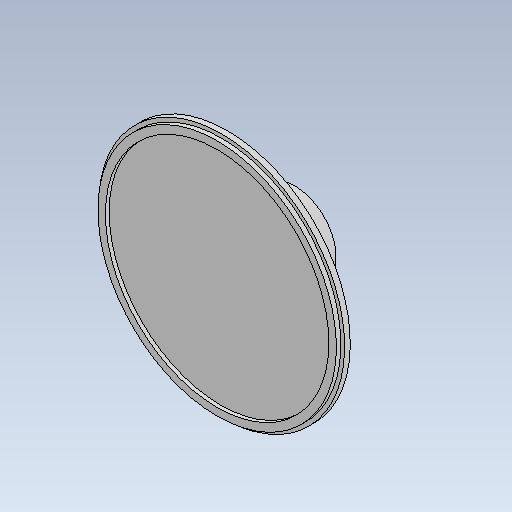
# Autodesk Inventor part: speaker
Saved by Autodesk Inventor 2026.1 (Build 301233020, 233B)
## iProperties
Created: 2026-08-11
Part Number: speaker
Material: 一般
Document SubType Name: Modeling
Designer: ug_nd
Density: 1 g/cm^3
Appearance: 既定
Author: ug_nd
Autodesk Inventor part; units mm, degrees
ref_plane "YZ Plane" through (0, 0, 0) normal (1, 0, 0) x (0, 1, 0)
ref_plane "XZ Plane" through (0, 0, 0) normal (0, 1, 0) x (-1, 0, 0)
sketch "スケッチ1" plane through (0, 0, 0) normal (1, 0, 0) x (0, 1, 0)
  line L0 (32.75, 0) -> (32.75, -1.5)
  line L1 (0, -23.64) -> (0, 5.34) construction
  line L2 (-6.55, 0) -> (39.3, 0) construction
  line L3 (32.75, -1.5) -> (30.25, -1.5)
  line L4 (30.25, -1.5) -> (30.25, -2.5)
  line L5 (30.25, -2.5) -> (17.5, -11.5)
  line L6 (17.5, -11.5) -> (11, -11.5)
  line L7 (32.75, 0) -> (31.75, 0)
  line L8 (31.75, 0) -> (31.75, 1.2)
  line L9 (11, -11.5) -> (11, -19.5)
  line L10 (11, -19.5) -> (0, -19.5)
  line L11 (0, -19.5) -> (0, 0.2)
  line L12 (31.75, 1.2) -> (29.75, 1.2)
  line L13 (29.75, 1.2) -> (29.75, 0.2)
  line L14 (29.75, 0.2) -> (0, 0.2)
  point P0 (0, 0)
  dimension "d0" = 65.5
  dimension "d1" = 1.5
  dimension "d2" = 60.5
  dimension "d3" = 35
  dimension "d4" = 1.2
  dimension "d5" = 63.5
  dimension "d7" = 11.5
  dimension "d8" = 1
  dimension "d9" = 22
  dimension "d10" = 8
  dimension "d11" = 59.5
  dimension "d12" = 1
  constraints: 26 end point, 6 horizontal, 6 vertical, 2 point on line
  measures "d0" diameter of L0 L1
  measures "d1" distance of L0.start L0.end
  measures "d2" diameter of L4 L1
  measures "d3" diameter of L5.end L1
  measures "d4" distance from line of L7 L8.end
  measures "d5" diameter of L8 L1
  measures "d7" distance between parallel lines of L7 L6
  measures "d8" distance from line of L3 L4.end
  measures "d9" diameter of L9 L1
  measures "d10" distance from line of L9.end L6
  measures "d11" diameter of L12.end L1
  measures "d12" distance between parallel lines of L12 L14
revolve "回転1" add sketch "スケッチ1" angle 360 about axis through (0, 0, -10) along (0, 0, 1)
sketch "スケッチ2" plane through (0, 0, -11.5) normal (0, 0, -1) x (-1, 0, 0)
  circle A0 centre (0, 0) radius 19 construction
  circle A1 centre (0, 0) radius 27.5 construction
  line L0 (-6, 26.837474) -> (-6, 18.027756)
  line L1 (45.85, 0) -> (-45.85, 0) construction
  line L2 (0, -45.85) -> (0, 45.85) construction
  line L3 (6, 26.837474) -> (6, 18.027756)
  arc A2 (-6, 26.837474) -> (-26.837474, 6) centre (0, 0) ccw
  arc A3 (-6, 18.027756) -> (-18.027756, 6) centre (0, 0) ccw
  line L4 (-26.837474, -6) -> (-18.027756, -6)
  arc A4 (-26.837474, -6) -> (-6, -26.837474) centre (0, 0) ccw
  arc A5 (-18.027756, -6) -> (-6, -18.027756) centre (0, 0) ccw
  line L5 (-26.837474, 6) -> (-18.027756, 6)
  line L6 (6, -26.837474) -> (6, -18.027756)
  arc A6 (6, -26.837474) -> (26.837474, -6) centre (0, 0) ccw
  arc A7 (6, -18.027756) -> (18.027756, -6) centre (0, 0) ccw
  line L7 (-6, -26.837474) -> (-6, -18.027756)
  line L8 (26.837474, 6) -> (18.027756, 6)
  arc A8 (26.837474, 6) -> (6, 26.837474) centre (0, 0) ccw
  arc A9 (18.027756, 6) -> (6, 18.027756) centre (0, 0) ccw
  line L9 (26.837474, -6) -> (18.027756, -6)
  point P0 (-6, -26.837474)
  point P1 (-6, -18.027756)
  point P2 (26.837474, -6)
  point P3 (18.027756, -6)
  point P4 (-26.837474, 6)
  point P5 (-18.027756, 6)
  dimension "d14" = 38
  dimension "d15" = 55
  dimension "d17" = 12
  dimension "d20" = 360
  constraints: 20 point on circle, 16 end point, 10 centre point, 4 coincident, 2 concentric, 2 symmetric about line, 1 vertical, 49 other
  measures "d14" diameter of A0
  measures "d15" diameter of A1
  measures "d17" distance between parallel lines of L3 L0
extrude "押し出し1" cut sketch "スケッチ2" against normal blind 8
fillet "フィレット1" radius 2 16 edges at (6, 26.8375, -3.9706) (6, 18.0278, -6.9706) (18.0278, 6, -6.9706) (26.8375, 6, -3.9706) (-6, 26.8375, -3.9706) (-6, 18.0278, -6.9706) (-18.0278, 6, -6.9706) (-26.8375, 6, -3.9706) (-26.8375, -6, -3.9706) (-18.0278, -6, -6.9706) (-6, -26.8375, -3.9706) (-6, -18.0278, -6.9706) (6, -18.0278, -6.9706) (6, -26.8375, -3.9706) (26.8375, -6, -3.9706) (18.0278, -6, -6.9706)
sketch "スケッチ3" plane through (0, 0, 0) normal (0, 0, 1) x (1, 0, 0)
  circle A0 centre (0, 0) radius 24
  dimension "d25" = 48
  constraints: 1 centre point, 1 coincident
  measures "d25" diameter of A0
sketch3d "3D スケッチ1"
ref_plane "作業平面1" through (0, -17.5, -11.5) normal (0, 0.5766832, 0.8169679) x (-1, 0, 0)
sketch "スケッチ4" plane through (0, -17.5, -11.5) normal (0, 0.5766832, 0.8169679) x (-1, 0, 0)
  line L0 (0, 0) -> (0, 15.606489) construction
  arc A0 (7.517645, 6.799173) -> (-7.517645, 6.799173) centre (0, -17.043751) ccw construction
  arc A1 (8.359621, 9.469581) -> (-8.359621, 9.469581) centre (0, -17.043751) ccw
  arc A2 (6.675669, 4.128766) -> (-6.675669, 4.128766) centre (0, -17.043751) ccw
  arc A3 (6.675669, 4.128766) -> (8.359621, 9.469581) centre (7.517645, 6.799173) ccw
  arc A4 (-8.359621, 9.469581) -> (-6.675669, 4.128766) centre (-7.517645, 6.799173) ccw
  ellipse E0 centre (0, -11.650979) end of major axis (-24, -11.650979) minor radius 19.607229 (6, 7.333638) -> (-6, 7.333638) ccw construction
  line L1 (0, -17.043751) -> (-7.517645, 6.799173) construction
  line L2 (0, -17.043751) -> (7.517645, 6.799173) construction
  circle A5 centre (-7.517645, 6.799173) radius 0.6
  circle A6 centre (7.517645, 6.799173) radius 0.6
  point P0 (0, -7.665081)
  point P1 (-27.923788, -10.053721)
  point P2 (-27.923788, -9.286433)
  point P3 (0, 7.956249)
  dimension "d30" = 2.8
  dimension "d33" = 25
  dimension "d34" = 35
  dimension "d37" = 1.2
  constraints: 11 point on circle, 7 centre point, 4 end point, 4 tangent, 2 coincident, 1 equal radius, 3 other
  measures "d30" radius of A3
  measures "d33" radius of A0
  measures "d34" angle of L2 L1
  measures "d37" diameter of A6
extrude "押し出し2" add sketch "スケッチ4" against normal blind 0.8
sketch "スケッチ5" plane through (0, -17.961347, -12.153574) normal (0, -0.5766832, -0.8169679) x (-1, 0, 0)
  circle A0 centre (-7.517645, -6.799173) radius 0.6
  line L0 (-7.517645, -6.799173) -> (-10.855654, -5.746703) construction
  arc A1 (-7.517645, -6.799173) -> (7.517645, -6.799173) centre (0, 17.043751) ccw construction
  circle A2 centre (-7.517645, -6.799173) radius 1.6
  circle A3 centre (-10.855654, -5.746703) radius 1.6
  arc A4 (-9.539441, -4.836987) -> (-8.074033, -5.299029) centre (-8.509435, -4.125088) ccw
  arc A5 (-8.833859, -7.708888) -> (-10.299267, -7.246847) centre (-9.863864, -8.420788) ccw
  line L1 (-8.885944, -5.319221) -> (-9.487355, -7.226655) construction
  circle A6 centre (-10.855654, -5.746703) radius 0.6
  point P0 (0, 7.665081)
  point P1 (-10.299267, -7.246847)
  point P2 (-8.833859, -7.708888)
  dimension "d39" = 3.2
  dimension "d38" = 3.5
  dimension "d40" = 2
  constraints: 6 point on circle, 4 end point, 4 symmetric about line, 3 centre point, 2 coincident, 1 tangent, 10 other
  measures "d38" distance of L0.start L0.end
  measures "d40" distance of L1.end L1.start
extrude "押し出し3" add sketch "スケッチ5" along normal blind 0.2
mirror "ミラー1" about plane through (0, 0, 0) normal (1, 0, 0) of "押し出し3"
